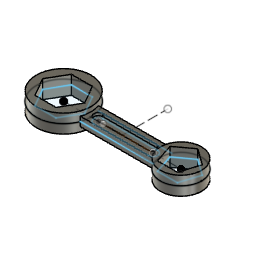
exercise 2 (Autodesk Fusion 360 design; units mm, degrees)
Autodesk Fusion 360 part; units mm, degrees
sketch "Sketch1" plane through (0, 0, 0) normal (0, 0, 1) x (1, 0, 0) in component "exercise 2"
  circle A0 centre (0, 0) radius 30
  line L0 (0, 0) -> (129, 0) construction
  circle A1 centre (129, 0) radius 22.5
  line L1 (28.2843, 10) -> (108.8444, 10)
  line L2 (28.2843, -10) -> (108.8444, -10)
  line L3 (-11.547, 20) -> (-23.094, 0)
  line L4 (-23.094, 0) -> (-11.547, -20)
  line L5 (-11.547, -20) -> (11.547, -20)
  line L6 (11.547, -20) -> (23.094, 0)
  line L7 (23.094, 0) -> (11.547, 20)
  line L8 (11.547, 20) -> (-11.547, 20)
  line L9 (140.0205, -14.9103) -> (146.5861, 5.8736)
  line L10 (146.5861, 5.8736) -> (128.8482, 18.5404)
  line L11 (128.8482, 18.5404) -> (111.3201, 5.585)
  line L12 (111.3201, 5.585) -> (118.225, -15.0887)
  line L13 (118.225, -15.0887) -> (140.0205, -14.9103)
  line L14 (64.5, 0) -> (64.5, 50) construction
  line L15 (38.2534, 0) -> (64.5, 0)
  line L16 (43.2534, 0) -> (98.2534, 0) construction
  line L17 (38.2534, 5) -> (98.2534, 5)
  line L18 (38.2534, -5) -> (98.2534, -5)
  arc A2 (38.2534, 5) -> (38.2534, -5) centre (38.2534, 0) ccw
  arc A3 (98.2534, -5) -> (98.2534, 5) centre (98.2534, 0) ccw
  point P0 (129, 0)
  dimension "d1" = 60
  dimension "d2" = 45
  dimension "d3" = 129
  dimension "d6" = 20
  dimension "d7" = 15
  dimension "d8" = 10
  dimension "d9" = 10
  dimension "d10" = 60
  constraint coincident A0.centre L0.start
  constraint coincident P0 L0.end
  constraint horizontal L0
  constraint coincident A1 L1.end
  constraint parallel L0 L1
  constraint coincident A1 L2.end
  constraint horizontal L2
  constraint midpoint L0 L14.start
  constraint perpendicular L1 L14
  constraint coincident L0 L15.start
  constraint coincident L0 L16.end
  constraint coincident L15.start A2.centre
  constraint coincident L16.end A3.centre
  constraint tangent L17 A2
  constraint tangent L17 A3
  constraint tangent L18 A2
  constraint tangent L18 A3
  constraint coincident A0 L1.start
  constraint coincident A0 L2.start
  measures "d1" diameter of A0
  measures "d2" diameter of A1
  measures "d3" distance of A0.centre P0
  measures "d6" distance of A0.centre L8
  measures "d7" distance of P0 L13
  measures "d8" diameter of A2
  measures "d9" diameter of A3
  measures "d10" distance of L15.start L16.end
extrude "Extrude1" add sketch "Sketch1" along normal mid plane 20 contours A0 | A1 makes body 1 at (27.1662, -12.7278, 3.3333) makes body 2 at (151.3882, -2.2403, -3.3333) in component "exercise 2"
extrude "Extrude2" add sketch "Sketch1" along normal mid plane 10 contours A0 A1 L1 L2 bodies 1 2 in component "exercise 2"
extrude "Extrude3" add sketch "Sketch1" along normal mid plane 4 contours L17 L18 A2 A3 bodies 1 in component "exercise 2"
component "exercise 2" placed x (1, 0, 0) y (0, 1, 0) z (0, 0, 1) at (0, 0, 0)
